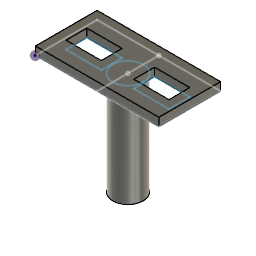
rod (Autodesk Fusion 360 design; units mm, degrees)
part number: 2026-02-28-00-34-00-891
Autodesk Fusion 360 part; units mm, degrees
note: some values were not read from the file. Set by a fixed rule: which sketch regions a step uses.
sketch "Sketch1" plane through (0, 0, 0) normal (0, 0, 1) x (1, 0, 0)
  line L0 (0, 0) -> (60, 0)
  line L1 (60, 0) -> (60, 30)
  line L2 (60, 30) -> (0, 30)
  line L3 (0, 30) -> (0, 0)
  circle A0 centre (30, 15) radius 7.4
  line L4 (5, 20) -> (22.0948, 20)
  line L5 (22.0948, 20) -> (22.0948, 9.9085)
  line L6 (22.0948, 9.9085) -> (5, 9.9085)
  line L7 (5, 9.9085) -> (5, 20)
  line L8 (30, 30) -> (30, 0)
  line L9 (55, 9.9085) -> (55, 20)
  line L10 (55, 20) -> (37.9052, 20)
  line L11 (37.9052, 20) -> (37.9052, 9.9085)
  line L12 (37.9052, 9.9085) -> (55, 9.9085)
  dimension "d1" = 60
  dimension "d2" = 30
  dimension "d3" = 14.8
  constraint horizontal L0
  constraint vertical L1
  constraint horizontal L2
  constraint vertical L3
  constraint coincident L0.start L3.end
  constraint horizontal L4
  constraint vertical L5
  constraint horizontal L6
  constraint vertical L7
  constraint midpoint L0 L8.end
  constraint perpendicular L0 L8
  constraint symmetric L4.start L8 L9.end
  constraint symmetric L4.end L8 L10.end
  constraint symmetric L5.end L8 L11.end
  constraint symmetric L6.end L8 L9.start
  measures "d1" distance of L0.start L0.end
  measures "d2" distance of L0.start L2.end
  measures "d3" diameter of A0
extrude "Extrude1" add sketch "Sketch1" along normal blind 4
extrude "Extrude2" add sketch "Sketch1" against normal blind 50 contours A0 L8 | A0 L8
